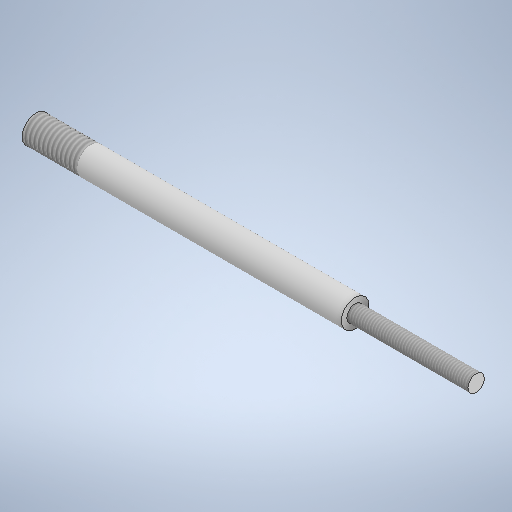
# Autodesk Inventor part: 19
Saved by Autodesk Inventor 2025.1 (Build 291241000, 241)
## iProperties
Created: 2024-09-17
Part Number: 19
Material: Generisch
Document SubType Name: Modeling
Designer: ffogue
Density: 1 g/cm^3
Appearance: Vorgabe
Author: ffogue
Autodesk Inventor part; units mm, degrees
ref_plane "YZ Plane" through (0, 0, 0) normal (1, 0, 0) x (0, 1, 0)
ref_plane "XZ Plane" through (0, 0, 0) normal (0, 1, 0) x (-1, 0, 0)
ref_plane "XY Plane" through (0, 0, 0) normal (0, 0, 1) x (1, 0, 0)
sketch "Sketch1" plane through (0, 0, 0) normal (0, 0, 1) x (1, 0, 0)
  line L0 (0, 0) -> (0, 2.5)
  line L1 (0, 2.5) -> (58, 2.5)
  line L2 (58, 2.5) -> (58, 1.5)
  line L3 (58, 1.5) -> (80, 1.5)
  line L4 (80, 1.5) -> (80, 0)
  line L5 (80, 0) -> (0, 0)
  dimension "d0" = 58
  dimension "d1" = 22
  dimension "d2" = 3
  dimension "d3" = 5
  constraints: 12 end point, 5 perpendicular, 1 vertical
  measures "d0" distance of L0.end L1.end
  measures "d1" distance of L2.end L3.end
  measures "d2" diameter of L3 L5
  measures "d3" diameter of L1 L5
revolve "Revolution1" add sketch "Sketch1" angle 360 about axis through (80, 0, 0) along (-1, 0, 0)
thread "Thread1" size "M3x0.5" class "6g" standard "ISO Metric profile" length 22
thread "Thread2" size "M5x0.8" class "6g" standard "ISO Metric profile" length 10
body "Solid1"
